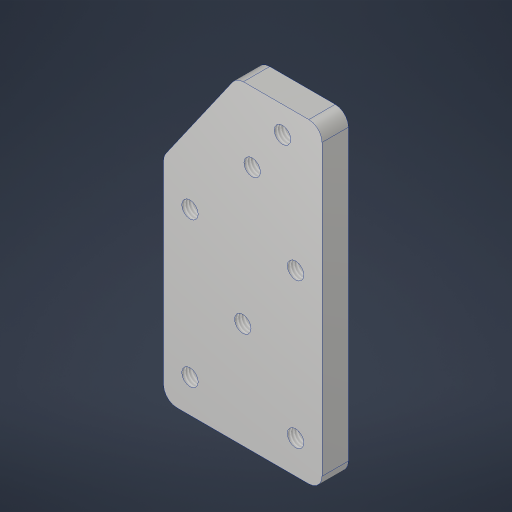
# Autodesk Inventor part: CL7-012
Saved by Autodesk Inventor 2023.4 (Build 274418000, 418)
## iProperties
Created: 2025-03-18
Part Number: CL7-012
Material: Aluminum 6061
Document SubType Name: Modeling
Designer: brand
Density: 2.7 g/cm^3
Appearance: Aluminum - Flat
Author: brand
Autodesk Inventor part; units mm, degrees
ref_plane "YZ Plane" through (0, 0, 0) normal (1, 0, 0) x (0, 1, 0)
ref_plane "XZ Plane" through (0, 0, 0) normal (0, 1, 0) x (-1, 0, 0)
ref_plane "XY Plane" through (0, 0, 0) normal (0, 0, 1) x (1, 0, 0)
sketch "Sketch1" plane through (0, 0, 0) normal (0, 0, 1) x (1, 0, 0)
  line L0 (0, 0) -> (355.6, 0) construction
  line L1 (355.6, 0) -> (355.6, 50.8) construction
  line L2 (355.6, 50.8) -> (0, 50.8) construction
  line L3 (0, 50.8) -> (0, 0) construction
  line L4 (57.1297, 50.8) -> (304.8, 404.5099) construction
  line L5 (304.8, 404.5099) -> (325.6065, 389.941) construction
  line L6 (325.6065, 389.941) -> (77.9362, 36.2312) construction
  line L7 (77.9362, 36.2312) -> (57.1297, 50.8) construction
  line L8 (355.6, 50.8) -> (304.8, 50.8) construction
  line L9 (304.8, 50.8) -> (304.8, 438.15) construction
  line L10 (304.8, 438.15) -> (355.6, 438.15) construction
  line L11 (355.6, 438.15) -> (355.6, 50.8) construction
  line L12 (57.15, 75.8737) -> (95.25, 75.8737)
  line L13 (95.25, 75.8737) -> (95.25, 0)
  line L14 (95.25, 0) -> (57.15, 0)
  line L15 (57.15, 0) -> (57.15, 75.8737)
  line L16 (320.675, 41.275) -> (288.925, 41.275) construction
  line L17 (288.925, 41.275) -> (288.925, 9.525) construction
  line L18 (288.925, 9.525) -> (320.675, 9.525) construction
  line L19 (320.675, 9.525) -> (320.675, 41.275) construction
  line L20 (234.95, 41.275) -> (203.2, 41.275) construction
  line L21 (203.2, 41.275) -> (203.2, 9.525) construction
  line L22 (203.2, 9.525) -> (234.95, 9.525) construction
  line L23 (234.95, 9.525) -> (234.95, 41.275) construction
  line L24 (67.5329, 43.5156) -> (111.2395, 105.935) construction
  circle A0 centre (63.5, 42.8625) radius 2.5527 construction
  line L25 (74.6865, 75.8737) -> (57.1297, 50.8)
  point P0 (88.1374, 50.8)
  point P1 (342.9, 42.8625)
  point P2 (330.2, 25.4)
  point P3 (342.9, 7.9375)
  point P4 (355.6, 25.4)
  point P5 (317.5, 42.8625)
  point P6 (304.8, 25.4)
  point P7 (317.5, 7.9375)
  point P8 (292.1, 42.8625)
  point P9 (279.4, 25.4)
  point P10 (292.1, 7.9375)
  point P11 (266.7, 42.8625)
  point P12 (254, 25.4)
  point P13 (266.7, 7.9375)
  point P14 (241.3, 42.8625)
  point P15 (228.6, 25.4)
  point P16 (241.3, 7.9375)
  point P17 (215.9, 42.8625)
  point P18 (203.2, 25.4)
  point P19 (215.9, 7.9375)
  point P20 (190.5, 42.8625)
  point P21 (177.8, 25.4)
  point P22 (190.5, 7.9375)
  point P23 (165.1, 42.8625)
  point P24 (152.4, 25.4)
  point P25 (165.1, 7.9375)
  point P26 (139.7, 42.8625)
  point P27 (127, 25.4)
  point P28 (139.7, 7.9375)
  point P29 (114.3, 42.8625)
  point P30 (101.6, 25.4)
  point P31 (114.3, 7.9375)
  point P32 (88.9, 42.8625)
  point P33 (76.2, 25.4)
  point P34 (88.9, 7.9375)
  point P35 (50.8, 25.4)
  point P36 (63.5, 7.9375)
  point P37 (38.1, 42.8625)
  point P38 (25.4, 25.4)
  point P39 (38.1, 7.9375)
  point P40 (12.7, 42.8625)
  point P41 (0, 25.4)
  point P42 (12.7, 7.9375)
  point P43 (-12.7, 42.8625)
  point P44 (-25.4, 25.4)
  point P45 (-12.7, 7.9375)
  point P46 (320.675, 25.4)
  point P47 (234.95, 25.4)
  point P48 (288.925, 25.4)
  point P49 (78.4596, 59.1204)
  point P50 (85.744, 69.5237)
  point P51 (93.0284, 79.9269)
  point P52 (100.3128, 90.3301)
  point P53 (57.15, 50.829)
  dimension "d0" = 50.8
  dimension "d1" = 355.6
  dimension "d2" = 55
  dimension "d3" = 25.4
  dimension "d4" = 50.8
  dimension "d5" = 387.35
  dimension "d6" = 431.8
  dimension "d10" = 12.7
  dimension "d11" = 7.9375
  dimension "d12" = 25.4
  dimension "d13" = 7.9375
  dimension "d16" = 25.4
  dimension "d21" = 34.925
  dimension "d22" = 31.75
  dimension "d23" = 31.75
  dimension "d24" = 31.75
  dimension "d25" = 120.65
  dimension "d26" = 31.75
  dimension "d27" = 76.2
  dimension "d28" = 19.05
  dimension "d31" = 12.7
  dimension "d37" = 6.35
  dimension "d38" = 6.35
  dimension "d39" = 6.35
  dimension "d40" = 5.1054
  constraints: 52 end point, 12 parallel, 8 point on line, 7 perpendicular, 6 horizontal, 5 midpoint, 3 horizontal alignment, 1 centre point, 1 coincident, 1 collinear, 1 vertical alignment, 46 other
  measures "d0" distance of L2.end L0.start
  measures "d1" distance of L0.start L0.end
  measures "d2" angle of L2 L6
  measures "d3" distance of L6.end L4.start
  measures "d4" distance of L9.end L10.end
  measures "d5" distance of L10.end L1.end
  measures "d6" distance of L4.start L4.end
  measures "d10" distance from line of L1 point (342.9, 42.863)
  measures "d11" distance from line of L2 point (342.9, 42.863)
  measures "d12" distance from line of L1 point (330.2, 25.4)
  measures "d13" distance from line of L0 point (342.9, 7.937)
  measures "d16" distance of point (342.9, 42.863) point (317.5, 42.863)
  measures "d21" distance between parallel lines of L1 L19
  measures "d22" distance of L16.start L16.end
  measures "d23" distance of L16.end L17.end
  measures "d24" distance of L21.end L22.end
  measures "d25" distance between parallel lines of L1 L23
  measures "d26" distance of L20.end L21.end
  measures "d27" distance of L24.start L24.end
  measures "d28" distance from line of point (78.46, 59.12) L7
  measures "d31" distance of point (78.46, 59.12) point (85.744, 69.524)
  measures "d37" distance from line of L13 point (88.9, 42.863)
  measures "d38" distance from line of L15 point (63.5, 42.863)
  measures "d39" distance from line of L12 point (85.744, 69.524)
  measures "d40" diameter of A0
extrude "Extrusion1" add sketch "Sketch1" against normal blind 6.35 contours L12 L13 L14 L15 L25
hole "Hole1" at (342.9, 42.8625, 0) at (330.2, 25.4, 0) at (342.9, 7.9375, 0) at (317.5, 42.8625, 0) at (304.8, 25.4, 0) at (317.5, 7.9375, 0) at (292.1, 42.8625, 0) at (279.4, 25.4, 0) at (292.1, 7.9375, 0) at (266.7, 42.8625, 0) at (254, 25.4, 0) at (266.7, 7.9375, 0) at (241.3, 42.8625, 0) at (228.6, 25.4, 0) at (241.3, 7.9375, 0) at (215.9, 42.8625, 0) at (203.2, 25.4, 0) at (215.9, 7.9375, 0) at (190.5, 42.8625, 0) at (177.8, 25.4, 0) at (190.5, 7.9375, 0) at (165.1, 42.8625, 0) at (152.4, 25.4, 0) at (165.1, 7.9375, 0) at (139.7, 42.8625, 0) at (127, 25.4, 0) at (139.7, 7.9375, 0) at (114.3, 42.8625, 0) at (101.6, 25.4, 0) at (114.3, 7.9375, 0) at (88.9, 42.8625, 0) at (76.2, 25.4, 0) at (88.9, 7.9375, 0) at (63.5, 42.8625, 0) at (50.8, 25.4, 0) at (63.5, 7.9375, 0) at (38.1, 42.8625, 0) at (25.4, 25.4, 0) at (38.1, 7.9375, 0) at (12.7, 42.8625, 0) at (0, 25.4, 0) at (12.7, 7.9375, 0) at (-12.7, 42.8625, 0) at (-25.4, 25.4, 0) at (-12.7, 7.9375, 0) at (78.4596, 59.1204, 0) at (85.744, 69.5237, 0) at (93.0284, 79.9269, 0) at (100.3128, 90.3301, 0) direction (0, 0, -1) diameter 3.9624 end through all thread size "10-32 UNF" class "2B" standard "ANSI Unified Screw Threads"
fillet "Fillet1" radius 3.175 5 edges at (57.15, 0, -3.175) (95.25, 0, -3.175) (57.15, 50.829, -3.175) (74.6865, 75.8737, -3.175) (95.25, 75.8737, -3.175)
equation "\"d13\" = d11"
equation "\"d23\" = d22"
equation "\"d24\" = d22"
equation "\"d26\" = d22"
equation "\"d38\" = d37"
equation "\"d39\" = d37"
body "Solid1"
